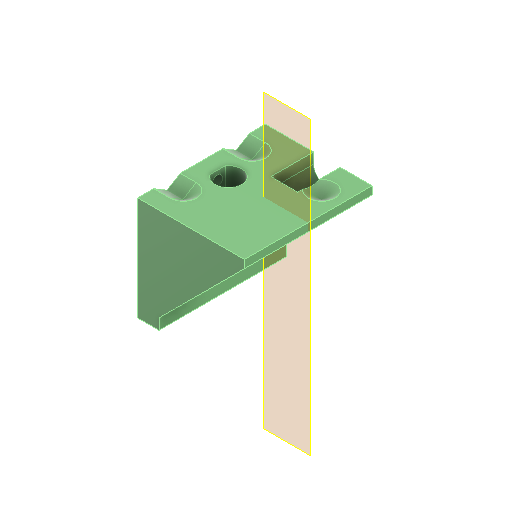
# Autodesk Inventor part: 20_Cube_Insert_Autofocus_KES400a_mirrorinsert_mirrorholder
Saved by Autodesk Inventor 2022 (Build 260153000, 153)
## iProperties
Created: 2023-06-13
Part Number: 20_Cube_Insert_Autofocus_KES400a_mirrorinsert_mirrorholder
Material: Generisch
Document SubType Name: Modeling
Designer: diederichbenedict
Density: 1 g/cm^3
Appearance: Glatt - Waldgrün
Author: diederichbenedict
Autodesk Inventor part; units mm, degrees
ref_plane "YZ Plane" through (0, 0, 0) normal (1, 0, 0) x (0, 1, 0)
ref_plane "XZ Plane" through (0, 0, 0) normal (0, 1, 0) x (-1, 0, 0)
ref_plane "XY Plane" through (0, 0, 0) normal (0, 0, 1) x (1, 0, 0)
ref_plane "Arbeitsebene1" through (25.7, 0, 0) normal (0, 0, 1) x (1, 0, 0)
sketch "Skizze1" plane through (25.7, 0, 0) normal (0, 0, 1) x (1, 0, 0)
  line L0 (-24, 30.5) -> (-24, 3.5) projected
  line L1 (-24, 30.5) -> (-4, 30.5) projected
  line L2 (-4, 30.5) -> (-4, 3.5) projected
  line L3 (-24, 3.5) -> (-4, 3.5) projected
  line L4 (-9.5, -19.9) -> (-9.5, 4.5)
  line L5 (-16.5, -19.9) -> (-16.5, 4.5)
  line L6 (-30.84, 17) -> (5.14, 17) construction
  line L7 (-20.0563, 9.7937) -> (-4.5, 25.35)
  line L8 (-20.0563, 9.7937) -> (1.9437, 9.7937) construction
  line L9 (-12.85, -15.6521) -> (-12.85, 34.845) construction
  line L10 (-4.5, 25.35) -> (-4.5, 27.35)
  line L11 (-4.5, 27.35) -> (-20.0563, 27.35)
  line L12 (-20.0563, 27.35) -> (-20.0563, 9.7937)
  line L13 (-20.0563, 9.7937) -> (-20.0563, 7.7937)
  line L14 (-20.0563, 7.7937) -> (-21.0563, 7.7937)
  line L15 (-21.0563, 7.7937) -> (-21.0563, 27.35)
  line L16 (-21.0563, 27.35) -> (-20.0563, 27.35)
  line L17 (-4.5, 27.35) -> (-3.5, 27.35)
  line L18 (-3.5, 27.35) -> (-3.5, 26.35)
  line L19 (-3.5, 26.35) -> (-4.5, 25.35)
  point P0 (-25.7, 0)
  point P1 (-12.85, 17)
  point P2 (-12.85, 17)
  point P3 (-20, 27.35)
  point P4 (-20, 9.85)
  point P5 (-4, 25.85)
  point P6 (-4, 27.35)
  dimension "d0" = 22
  dimension "d1" = 45
  dimension "d2" = 3.35
  dimension "d3" = 0.5
  dimension "d4" = 2
  dimension "d7" = 2
  dimension "d8" = 1
  dimension "d29" = 1
  constraints: 32 end point, 6 perpendicular, 5 vertical, 3 horizontal, 2 midpoint, 2 point on line, 1 equal length, 7 other
  measures "d0" distance of L7.start L7.end
  measures "d1" angle of L8 L7
  measures "d2" distance between parallel lines of L4 L9
  measures "d3" distance from line of L7.end L2
  measures "d4" distance of L7.end L10.end
  measures "d7" distance of L7.start L13.end
  measures "d8" distance of L13.end L14.end
  measures "d29" distance of L10.end L17.end
extrude "Extrusion1" add sketch "Skizze1" along normal mid plane 24 contours L2 L19 L10 L17 | L10 L7 L12 L11 | L12 L13 L14 L15 L16
sketch "Skizze3" plane through (4.6437, 7.7937, 12) normal (-1, 0, 0) x (0, 0, 1)
  arc A0 (-2, 12.6705) -> (-14, 19.5987) centre (-10, 12.6705) ccw projected
  line L0 (-2, 5.7422) -> (-2, 12.6705) projected
  arc A1 (-14, -1.186) -> (-2, 5.7422) centre (-10, 5.7422) ccw projected
  line L1 (-20, 2.2781) -> (-14, -1.186) projected
  arc A2 (-20, 16.1346) -> (-20, 2.2781) centre (-16, 9.2063) ccw projected
  line L2 (-14, 19.5987) -> (-20, 16.1346) projected
  line L3 (-25.5, 22.7063) -> (1.5, 22.7063) projected
  line L4 (-25.5, -4.2937) -> (-25.5, 22.7063) projected
  line L5 (1.5, -4.2937) -> (-25.5, -4.2937) projected
  line L6 (1.5, 22.7063) -> (1.5, -4.2937) projected
  circle A3 centre (-12, 9.7063) radius 6
  point P0 (-12, -7.7937)
  dimension "d16" = 12
  constraints: 1 centre point
  measures "d16" diameter of A3
extrude "Extrusion2" cut sketch "Skizze3" against normal blind 24 contours A3
sketch "Skizze4" plane through (21.2, 25.35, 12) normal (0.7071068, -0.7071068, 0) x (-0.7071068, -0.7071068, 0)
  ellipse E0 centre (11.1016, 12) end of major axis (19.5869, 12) minor radius 6 projected
  line L0 (20.6016, 21.5) -> (1.6016, 21.5)
  line L1 (1.6016, 21.5) -> (1.6016, 2.5)
  line L2 (1.6016, 2.5) -> (20.6016, 2.5)
  line L3 (20.6016, 2.5) -> (20.6016, 21.5)
  line L4 (20.6016, 21.5) -> (1.6016, 2.5) construction
  line L5 (1.6016, 21.5) -> (20.6016, 2.5) construction
  point P0 (32.9158, 12)
  dimension "d19" = 19
  dimension "d20" = 19
  constraints: 12 end point, 2 midpoint, 2 parallel, 1 coincident, 1 horizontal, 1 perpendicular
  measures "d19" distance of L2.end L1.end
  measures "d20" distance of L1.end L0.end
extrude "Extrusion3" cut sketch "Skizze4" against normal blind 0.5 contours E0 | L3 L2 L1 L0
sketch "Skizze8" plane through (4.6437, 27.35, 12) normal (0, 1, 0) x (1, 0, 0)
  line L0 (-2.4437, -5) -> (-2.4437, 13.6583) projected
  line L1 (-2.4437, -5) -> (20.5563, -5) projected
  line L2 (20.5563, 29) -> (20.5563, 13.5706) projected
  line L3 (-2.4437, 29) -> (4.3112, 29) projected
  line L4 (-2.4437, 13.6583) -> (-2.4437, 29) projected
  circle A0 centre (0.0563, 5.5) radius 1.4 projected
  circle A1 centre (13.0563, 18.5) radius 1.4 projected
  circle A2 centre (6.5563, 18.5) radius 3 projected
  circle A3 centre (0.0563, 18.5) radius 1.4 projected
  arc A4 (-2.4437, 10.3417) -> (-2.4437, 13.6583) centre (0.0563, 12) ccw projected
  line L5 (20.5563, 10.4294) -> (17.0563, 10.4294) projected
  line L6 (17.0563, 10.4294) -> (17.0563, 13.5706) projected
  line L7 (17.0563, 13.5706) -> (20.5563, 13.5706) projected
  line L8 (8.8015, 29) -> (20.5563, 29) projected
  line L9 (8.8015, 29) -> (8.8015, 25) projected
  line L10 (8.8015, 25) -> (4.3112, 25) projected
  line L11 (4.3112, 25) -> (4.3112, 29) projected
  line L12 (20.5563, 10.4294) -> (20.5563, -5) projected
  point P0 (-4.6437, 12)
hole "Bohrung2" at (4.7, 27.35, -6.5) at (17.7, 27.35, -6.5) at (4.7, 27.35, 6.5) direction (0, -1, 0) diameter 5 depth 0.01 tip angle 118
sketch "Skizze9" plane through (25.7, 0, -12) normal (0, 0, -1) x (-1, 0, 0)
  line L0 (15, 41.9) -> (15, 29.5)
  line L1 (23.5, 34) -> (0.5, 34) projected
  line L2 (10, 41.9) -> (10, 29.5)
  line L3 (21.0563, 27.35) -> (4, 27.35) projected
  line L4 (15, 27.35) -> (10, 27.35)
  line L5 (10, 27.35) -> (10, 25.35)
  line L6 (10, 25.35) -> (15, 25.35)
  line L7 (15, 25.35) -> (15, 27.35)
  arc A0 (10, 25.35) -> (15, 25.35) centre (12.5, 25.35) ccw
  point P0 (25.7, 0)
  point P1 (10, 27.35)
  dimension "d39" = 2
  constraints: 12 end point, 2 parallel, 2 point on circle, 2 tangent, 2 vertical, 1 centre point, 1 horizontal, 1 perpendicular, 1 point on line, 4 other
  measures "d39" distance of L5.end L4.end
extrude "Extrusion7" cut sketch "Skizze9" against normal blind 8
sketch "Skizze10" plane through (25.7, 0, -4) normal (0, 0, -1) x (-1, 0, 0)
  arc A0 (10, 25.35) -> (15, 25.35) centre (12.5, 25.35) ccw projected
  circle A1 centre (12.5, 25.35) radius 0.95
  point P0 (25.7, 0)
  dimension "d42" = 1.9
  constraints: 1 centre point, 1 coincident
  measures "d42" diameter of A1
extrude "Extrusion8" cut sketch "Skizze10" against normal blind 8
sketch "Skizze11" plane through (4.6437, 27.35, 12) normal (0, 1, 0) x (1, 0, 0)
  circle A0 centre (2.0563, 12) radius 2.5
  arc A1 (-2.4437, 10.3417) -> (-2.4437, 13.6583) centre (0.0563, 12) ccw projected
  point P0 (-4.6437, 12)
  dimension "d45" = 5
  constraints: 1 centre point
  measures "d45" diameter of A0
extrude "Extrusion9" cut sketch "Skizze11" against normal blind 8
sketch "Skizze12" plane through (4.6437, 7.7937, -12) normal (-1, 0, 0) x (0, 0, 1)
  line L0 (9.5, 19.5563) -> (9.5, 15.1607) projected
  line L1 (14.5, 19.5563) -> (14.5, 15.1607) projected
  circle A0 centre (12, 17.8198) radius 0.95
  point P0 (12, -7.7937)
  dimension "d48" = 1.9
  constraints: 1 centre point
  measures "d48" diameter of A0
extrude "Extrusion10" cut sketch "Skizze12" against normal blind 8
sketch "Skizze13" plane through (4.6437, 7.7937, -12) normal (-1, 0, 0) x (0, 0, 1)
  line L0 (7.9994, 19.5563) -> (7.9994, 19.5463) projected
  spline S0 degree 2 poles (7.9994, 19.5463) (5.5, 18.045) (3.0006, 19.5463) knots 0 0 0 1 1 1 weights 1 44.366213 1 projected
  line L1 (3.0006, 19.5463) -> (3.0006, 19.5563) projected
  line L2 (3.0006, 19.5563) -> (0, 19.5563) projected
  line L3 (0, 0) -> (0, 19.5563) projected
  line L4 (0, 0) -> (24, 0) projected
  line L5 (24, 19.5563) -> (24, 0) projected
  line L6 (24, 19.5563) -> (20.9994, 19.5563) projected
  line L7 (20.9994, 19.5563) -> (20.9994, 19.5463) projected
  spline S1 degree 2 poles (20.9994, 19.5463) (18.5, 18.045) (16.0006, 19.5463) knots 0 0 0 1 1 1 weights 1 44.366213 1 projected
  line L8 (16.0006, 19.5463) -> (16.0006, 19.5563) projected
  line L9 (16.0006, 19.5563) -> (13.4218, 19.5563) projected
  arc A0 (10.5782, 15.5355) -> (13.4218, 15.5355) centre (12, 9.7063) ccw projected
  line L10 (13.4218, 19.5563) -> (13.4218, 15.5355) projected
  line L11 (10.5782, 15.5355) -> (10.5782, 19.5563) projected
  line L12 (10.5782, 19.5563) -> (7.9994, 19.5563) projected
  line L13 (13.4218, 19.5563) -> (13.4218, 15.5355) projected
  line L14 (10.5782, 15.5355) -> (10.5782, 19.5563) projected
  arc A1 (13.4218, 15.5355) -> (10.5782, 15.5355) centre (12, 9.7063) ccw
  line L15 (9.5, 19.5563) -> (14.5, 19.5563) projected
  spline S2 degree 2 poles (12.95, 17.8198) (12.95, 19.4652) (11.525, 18.6425) (10.1, 17.8198) (11.525, 16.9971) (12.95, 16.1743) (12.95, 17.8198) knots 0 0 0 0.333333 0.333333 0.666667 0.666667 1 1 1 weights 1 0.5 1 0.5 1 0.5 1 projected
  point P0 (12, -7.7937)
  constraints: 2 horizontal alignment, 2 point on circle, 1 centre point, 1 other
extrude "Extrusion11" add sketch "Skizze13" along normal blind 3 contours L12 L11 A0 L10 L9 L8 S1 L7 L6 L5 L4 L3 L2 L1 S0 L0 | L15 L10 A1 L11
